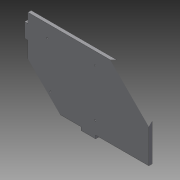
# Autodesk Inventor part: Center_Mount
Saved by Autodesk Inventor 2014 (Build 180170000, 170)
## iProperties
Created: 2015-02-09
Part Number: Center_Mount
Material: Generic
Document SubType Name: Modeling
Designer: ThatOtherGuy
Density: 1 g/cm^3
Appearance: Default
Author: ThatOtherGuy
Autodesk Inventor part; units mm, degrees
ref_plane "YZ Plane" through (0, 0, 0) normal (1, 0, 0) x (0, 1, 0)
ref_plane "XZ Plane" through (0, 0, 0) normal (0, 1, 0) x (-1, 0, 0)
ref_plane "XY Plane" through (0, 0, 0) normal (0, 0, 1) x (1, 0, 0)
sketch "Sketch1" plane through (0, 0, 0) normal (0, 0, 1) x (1, 0, 0)
  line L0 (0, 0) -> (250, 0)
  line L1 (250, 0) -> (250, 150)
  line L2 (250, 150) -> (0, 150)
  line L3 (0, 150) -> (0, 0)
  dimension "d0" = 150
  dimension "d1" = 250
  constraints: 8 end point, 2 parallel, 1 horizontal, 1 perpendicular
  measures "d0" distance of L2.end L0.start
  measures "d1" distance of L0.start L0.end
extrude "Extrusion1" add sketch "Sketch1" along normal blind 6.731
sketch "Sketch2" plane through (0, 0, 6.731) normal (0, 0, 1) x (1, 0, 0)
  line L0 (0, 0) -> (250, 0) projected
  line L1 (250, 0) -> (250, 150) projected
  line L2 (250, 150) -> (0, 150) projected
  line L3 (0, 150) -> (0, 0) projected
  point P0 (72.455, 31.185)
  point P1 (65.47, 123.895)
  point P2 (164.53, 123.895)
  point P3 (164.53, 26.105)
  dimension "d4" = 92.075
  dimension "d5" = 5.08
  dimension "d6" = 92.71
  dimension "d7" = 6.985
  dimension "d8" = 26.105
  dimension "d9" = 26.105
  dimension "d10" = 65.47
  dimension "d11" = 85.47
  constraints: 1 horizontal alignment, 1 vertical alignment
  measures "d4" horizontal distance of point (72.455, 31.185) point (164.53, 26.105)
  measures "d5" vertical distance of point (72.455, 31.185) point (164.53, 26.105)
  measures "d6" vertical distance of point (65.47, 123.895) point (72.455, 31.185)
  measures "d7" horizontal distance of point (72.455, 31.185) point (65.47, 123.895)
  measures "d8" distance from line of L2 point (164.53, 123.895)
  measures "d9" distance from line of L0 point (164.53, 26.105)
  measures "d10" distance from line of L3 point (65.47, 123.895)
  measures "d11" distance from line of L1 point (164.53, 26.105)
hole "Hole1" at (72.455, 31.185, 6.731) at (65.47, 123.895, 6.731) at (164.53, 123.895, 6.731) at (164.53, 26.105, 6.731) direction (0, 0, -1) diameter 3.176 end through all
sketch "Sketch3" plane through (0, 0, 6.731) normal (0, 0, 1) x (1, 0, 0)
  line L0 (0, 0) -> (250, 0) projected
  line L1 (250, 0) -> (250, 150) projected
  line L2 (0, 150) -> (0, 0) projected
  line L3 (0, 100) -> (-6.731, 100)
  line L4 (-6.731, 100) -> (-6.731, 130)
  line L5 (-6.731, 130) -> (0, 130)
  line L6 (0, 130) -> (0, 100)
  line L7 (250, 130) -> (256.731, 130)
  line L8 (256.731, 130) -> (256.731, 100)
  line L9 (256.731, 100) -> (250, 100)
  line L10 (250, 100) -> (250, 130)
  line L11 (110, 0) -> (140, 0)
  line L12 (140, 0) -> (140, -6.731)
  line L13 (140, -6.731) -> (110, -6.731)
  line L14 (110, -6.731) -> (110, 0)
  line L15 (250, 150) -> (0, 150) projected
  line L16 (45, 150) -> (75, 150)
  line L17 (75, 150) -> (75, 156.731)
  line L18 (75, 156.731) -> (45, 156.731)
  line L19 (45, 156.731) -> (45, 150)
  line L20 (175, 150) -> (205, 150)
  line L21 (205, 150) -> (205, 156.731)
  line L22 (205, 156.731) -> (175, 156.731)
  line L23 (175, 156.731) -> (175, 150)
  line L24 (75, 156.731) -> (175, 156.731) construction
  point P0 (125, 0)
  point P1 (125, 0)
  point P2 (125, 156.731)
  point P3 (125, 150)
  dimension "d19" = 6.731
  dimension "d20" = 30
  dimension "d21" = 100
  dimension "d24" = 100
  constraints: 42 end point, 10 parallel, 8 equal length, 6 perpendicular, 5 horizontal, 5 point on line, 4 midpoint, 1 coincident, 1 collinear, 1 vertical alignment
  measures "d19" distance of L4.end L5.end
  measures "d20" distance of L3.end L4.end
  measures "d21" distance between parallel lines of L0 L3
  measures "d24" distance of L17.end L22.end
extrude "Extrusion2" add sketch "Sketch3" against normal up to surface (6.731 mm away) contours L0 L12 L13 L14 | L3 L4 L5 L2 | L1 L7 L8 L9 | L19 L18 L17 L15 | L23 L22 L21 L15
sketch "Sketch4" plane through (0, 0, 6.731) normal (0, 0, 1) x (1, 0, 0)
  line L0 (0, 0) -> (110, 0) projected
  line L1 (0, 100) -> (0, 0) projected
  line L2 (0, 50) -> (30, 50)
  line L3 (30, 50) -> (30, 0)
  dimension "d25" = 50
  dimension "d26" = 30
  constraints: 4 end point, 2 perpendicular, 1 midpoint, 1 point on line
  measures "d25" distance of L2.end L3.end
  measures "d26" distance of L2.start L2.end
extrude "Extrusion3" cut sketch "Sketch4" against normal up to next
equation "\"d2\" = THICKB"
equation "\"d8\" = d9"
equation "\"d19\" = THICKB"
equation "\"THICKA\" = 3.175"
equation "\"THICKB\" = 6.731"
equation "\"THICKC\" = 12.7"
equation "\"THICKPLY\" = 5"
equation "\"MAGDIA\" = 9.5"
equation "\"BALLDIA\" = 12"
body "Solid1"
